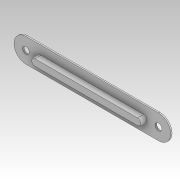
# Autodesk Inventor part: OldWankelBracket
Saved by Autodesk Inventor 2020 (Build 240168000, 168)
## iProperties
Created: 2022-01-26
Part Number: OldWankelBracket
Material: Generic
Document SubType Name: Modeling
Designer: DDeGo
Density: 1 g/cm^3
Appearance: Default
Author: DDeGo
Autodesk Inventor part; units mm, degrees
ref_plane "YZ Plane" through (0, 0, 0) normal (1, 0, 0) x (0, 1, 0)
ref_plane "XZ Plane" through (0, 0, 0) normal (0, 1, 0) x (-1, 0, 0)
ref_plane "XY Plane" through (0, 0, 0) normal (0, 0, 1) x (1, 0, 0)
sketch "Sketch1" plane through (0, 0, 0) normal (0, 0, 1) x (1, 0, 0)
  line L0 (-55, 0) -> (55, 0) construction
  line L1 (-55, -10) -> (55, -10)
  line L2 (55, 10) -> (-55, 10)
  arc A0 (-55, 10) -> (-55, -10) centre (-55, 0) ccw
  arc A1 (55, -10) -> (55, 10) centre (55, 0) ccw
  circle A2 centre (-55, 0) radius 2.75
  circle A3 centre (55, 0) radius 2.75
  point P0 (0, 0)
  dimension "d0" = 10
  dimension "d1" = 110
  dimension "d2" = 5.5
  constraints: 8 end point, 4 centre point, 4 point on circle, 4 tangent, 2 coincident, 1 equal radius, 1 horizontal, 1 midpoint, 1 parallel
  measures "d0" radius of A1
  measures "d1" distance of L0.start L0.end
  measures "d2" diameter of A2
extrude "Extrusion1" add sketch "Sketch1" along normal blind 1.1
sketch "Sketch2" plane through (0, 0, 1.1) normal (0, 0, 1) x (1, 0, 0)
  line L0 (42.5, 0) -> (-42.5, 0) construction
  line L1 (42.5, 2.75) -> (-42.5, 2.75)
  line L2 (-42.5, -2.75) -> (42.5, -2.75)
  arc A0 (42.5, -2.75) -> (42.5, 2.75) centre (42.5, 0) ccw
  arc A1 (-42.5, 2.75) -> (-42.5, -2.75) centre (-42.5, 0) ccw
  point P0 (0, 0)
  dimension "d5" = 5.5
  dimension "d6" = 85
  constraints: 8 end point, 4 point on circle, 4 tangent, 2 centre point, 1 horizontal, 1 midpoint, 1 parallel
  measures "d5" distance between parallel lines of L2 L1
  measures "d6" distance of L0.start L0.end
extrude "Extrusion2" add sketch "Sketch2" along normal blind 5
body "Solid1"
